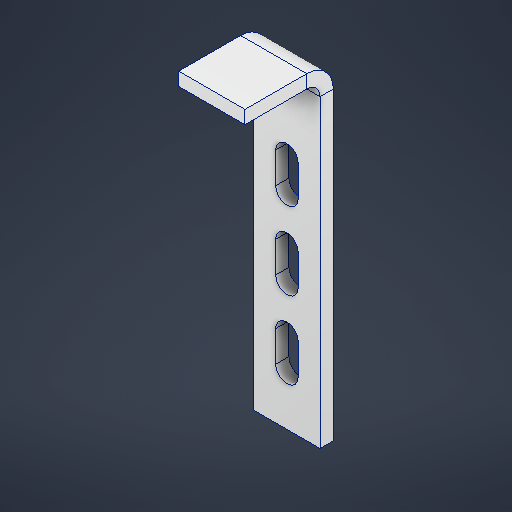
# Autodesk Inventor part: Support Bracket
Saved by Autodesk Inventor 2026 (Build 300175000, 175)
## iProperties
Created: 2025-11-03
Part Number: Support Bracket
Material: Aluminum 6061
Document SubType Name: Sheet Metal
Designer: Brandon Portillo
Density: 2.7 g/cm^3
Sheet Metal Rule: Default
Appearance: Aluminum - Flat
Author: Brandon Portillo
Autodesk Inventor part; units mm, degrees
ref_plane "YZ Plane" through (0, 0, 0) normal (1, 0, 0) x (0, 1, 0)
ref_plane "XZ Plane" through (0, 0, 0) normal (0, 1, 0) x (-1, 0, 0)
ref_plane "XY Plane" through (0, 0, 0) normal (0, 0, 1) x (1, 0, 0)
sketch "Sketch1" plane through (0, 0, 0) normal (0, 0, 1) x (1, 0, 0)
  line L0 (0, 0) -> (30, 0)
  line L1 (30, 0) -> (30, 150)
  line L2 (30, 150) -> (0, 150)
  line L3 (0, 150) -> (0, 0)
  dimension "d0" = 30
  dimension "d1" = 150
  measures "d0" distance of L2.end L1.end
  measures "d1" distance of L1.end L0.end
extrude "Plate1" add sketch "Sketch1" along normal blind 6
sketch "Sketch2" plane through (0, 144, 0) normal (0, 1, 0) x (-1, 0, 0)
  line L0 (-30, 0) -> (0, 0)
  line L1 (0, 0) -> (0, 40)
  line L2 (0, 40) -> (-30, 40)
  line L3 (-30, 40) -> (-30, 0)
  constraints: 6 end point, 1 horizontal, 1 perpendicular, 1 vertical
edge flange "Flange1" height 40 angle 90 thickness 6 bend radius 6 thickness toward (0, 1, 0) relief straight relief width 6 relief depth 3 edges at (15, 150, 6) wall of the first edge with corners at (30, 144, 0) (0, 144, 0) (0, 144, 40) (30, 144, 40)
bend "Bend1"
corner "Corner1"
sketch "Sketch3" plane through (0, 0, 6) normal (0, 0, 1) x (1, 0, 0)
  line L0 (30, 0) -> (0, 0) projected
  line L1 (15, 0) -> (15, 30)
  line L2 (15, 30) -> (15, 65)
  line L3 (15, 65) -> (15, 100)
  line L4 (15, 93) -> (15, 107) construction
  line L5 (20.1, 93) -> (20.1, 107)
  line L6 (9.9, 107) -> (9.9, 93)
  arc A0 (9.9, 93) -> (20.1, 93) centre (15, 93) ccw
  arc A1 (20.1, 107) -> (9.9, 107) centre (15, 107) ccw
  line L7 (15, 58) -> (15, 72) construction
  line L8 (20.1, 58) -> (20.1, 72)
  line L9 (9.9, 72) -> (9.9, 58)
  arc A2 (9.9, 58) -> (20.1, 58) centre (15, 58) ccw
  arc A3 (20.1, 72) -> (9.9, 72) centre (15, 72) ccw
  line L10 (15, 23) -> (15, 37) construction
  line L11 (20.1, 23) -> (20.1, 37)
  line L12 (9.9, 37) -> (9.9, 23)
  arc A4 (9.9, 23) -> (20.1, 23) centre (15, 23) ccw
  arc A5 (20.1, 37) -> (9.9, 37) centre (15, 37) ccw
  dimension "d13" = 30
  dimension "d14" = 35
  dimension "d15" = 35
  dimension "d16" = 7
  dimension "d17" = 10.2
  dimension "d18" = 7
  dimension "d19" = 10.2
  dimension "d20" = 7
  dimension "d21" = 10.2
  constraints: 30 end point, 12 point on circle, 12 tangent, 6 centre point, 5 point on line, 4 midpoint, 3 coincident, 3 parallel, 1 vertical
  measures "d13" distance of L1.start L1.end
  measures "d14" distance of L1.end L2.end
  measures "d15" distance of L2.end L3.end
  measures "d16" distance of point (15, 100) L4.end
  measures "d17" diameter of A1
  measures "d18" distance of point (15, 65) L7.end
  measures "d19" diameter of A3
  measures "d20" distance of point (15, 30) L10.end
  measures "d21" diameter of A5
extrude "Cut1" cut sketch "Sketch3" against normal blind 6
equation "\"d22\" = Thickness"
equation "\"d2\" = Thickness"
equation "\"d3\" = BendReliefWidth"
equation "\"d4\" = BendReliefDepth"
equation "\"d5\" = MinimumRemnant"
equation "\"d6\" = TransitionRadius"
equation "\"d9\" = BendRadius"
equation "\"d10\" = CornerReliefSize"
equation "\"d11\" = GapSize"
equation "\"d12\" = JacobiRadiusSize"
equation "\"BendRadius\" = Thickness"
equation "\"BendReliefWidth\" = Thickness"
equation "\"BendReliefDepth\" = 0.5 * Thickness"
equation "\"CornerReliefSize\" = 4 * Thickness"
equation "\"MinimumRemnant\" = 2 * Thickness"
equation "\"TransitionRadius\" = BendRadius"
equation "\"JacobiRadiusSize\" = BendRadius"
equation "\"GapSize\" = Thickness"
equation "\"Thickness\" = 6"
body "Solid1"
